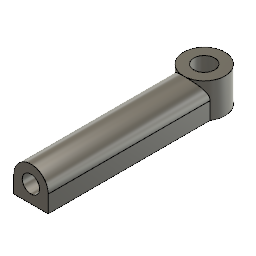
Agarre de palito (Autodesk Fusion 360 design; units mm, degrees)
Autodesk Fusion 360 part; units mm, degrees
note: some values were not read from the file. Chosen so that the rebuilt part matches the saved one: which bodies a step acts on; which pieces of a blend or face edit are solid.
sketch "Sketch1" plane through (0, 0, 0) normal (0, 1, 0) x (1, 0, 0)
  circle A0 centre (0, 0) radius 3
  circle A1 centre (0, 0) radius 6
  dimension "d1" = 6
  constraint coincident A0.centre A1.centre
  measures "d1" diameter of A0
extrude "Extrude1" add sketch "Sketch1" along normal blind 10 makes body 1
sketch "Sketch2" plane through (0, 0, 0) normal (0, 0, 1) x (1, 0, 0)
  line L0 (0, 0) -> (0, 5)
  circle A0 centre (0, 5) radius 2.5
  circle A1 centre (0, 5) radius 5
  dimension "d4" = 5
  dimension "d5" = 5
  dimension "d6" = 10
  constraint coincident L0.start origin
  constraint vertical L0
  constraint coincident L0.end A0.centre
  constraint concentric A0 A1
  measures "d4" distance of L0.start L0.end
  measures "d5" diameter of A0
  measures "d6" diameter of A1
extrude "Extrude2" add sketch "Sketch2" along normal blind 50 bodies 1
delete_face "DeleteFace1" 1 faces at (0, 10, 1) on bodies 1
sketch "Sketch3" plane through (0, 0, 0) normal (0, 1, 0) x (1, 0, 0)
  line L0 (5, -50) -> (-5, -50)
  line L1 (-5, -50) -> (-5, -3)
  line L2 (-5, -3) -> (5, -3)
  line L3 (5, -3) -> (5, -50)
  constraint horizontal L0
  constraint vertical L1
  constraint horizontal L2
  constraint vertical L3
extrude "Extrude3" add sketch "Sketch3" along normal blind 5 separate body makes body 2
copy_body "CopyPasteBodies2" bodies 1 makes body 3
combine "Combine1" operation cut target body 2 tool bodies 1 makes body 4 at (4.1903, 2.2721, 19.5362) makes body 4 at (-4.9858, 4.623, 34.4476)
combine "Combine2" operation add target body 4 tool bodies 3
hidden bodies 2
